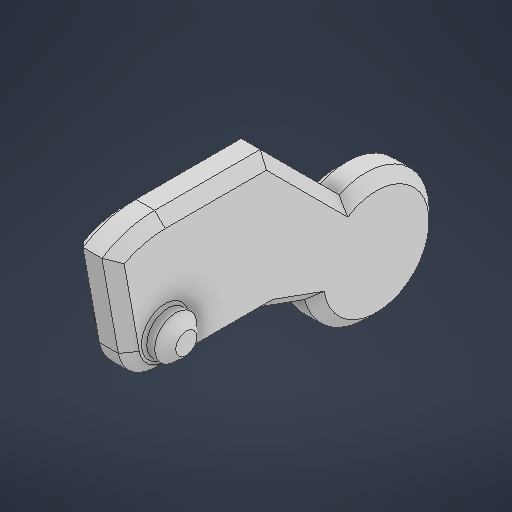
# Autodesk Inventor part: TrainPullert
Saved by Autodesk Inventor 2026.3 (Build 303398000, 398)
## iProperties
Created: 2026-05-02
Part Number: TrainPullert
Material: Generic
Document SubType Name: Modeling
Designer: frede
Density: 1 g/cm^3
Appearance: Default
Author: frede
Autodesk Inventor part; units mm, degrees
ref_plane "YZ Plane" through (0, 0, 0) normal (1, 0, 0) x (0, 1, 0)
ref_plane "XZ Plane" through (0, 0, 0) normal (0, 1, 0) x (-1, 0, 0)
ref_plane "XY Plane" through (0, 0, 0) normal (0, 0, 1) x (1, 0, 0)
sketch "Sketch1" plane through (0, 0, 0) normal (1, 0, 0) x (0, 1, 0)
  arc A0 (9.4, 0) -> (7.9599, 5) centre (0, 0) ccw
  circle A1 centre (0, 0) radius 3.5
  line L0 (-0.6243, 3.4439) -> (7.9599, 5)
  line L1 (-3.5, 0) -> (-3.5, -10)
  line L2 (9.4, 0) -> (9.4, -10)
  line L3 (-3.5, -10) -> (-5.0279, -14.1978)
  line L4 (-3.5, -10) -> (26.5, -10) construction
  line L5 (1.9372, -17.4628) -> (9.4, -10)
  arc A2 (-5.0279, -14.1978) -> (1.9372, -17.4628) centre (-3.5, -20) ccw
  dimension "d0" = 18.8
  dimension "d2" = 7
  dimension "d4" = 5
  dimension "d5" = 10
  dimension "d7" = 110
  dimension "d25" = 45
  dimension "d26" = 12
  constraints: 12 end point, 6 point on circle, 3 centre point, 3 tangent, 2 coincident, 2 vertical, 1 horizontal
  measures "d0" diameter of A0
  measures "d2" diameter of A1
  measures "d4" vertical distance of point (0, 0) L0.end
  measures "d5" distance of L2.start L2.end
  measures "d7" angle of L3 L4
  measures "d25" angle of L2 L5
  measures "d26" diameter of A2
extrude "Extrusion1" add sketch "Sketch1" along normal blind 3.8
sketch "Sketch2" plane through (3.8, 0, 0) normal (1, 0, 0) x (0, 0, -1)
  circle A0 centre (0, 0) radius 2
  dimension "d12" = 4
  constraints: 1 centre point, 1 coincident
  measures "d12" diameter of A0
extrude "Extrusion2" add sketch "Sketch2" along normal blind 2
sketch "Sketch3" plane through (0, 0, 0) normal (-1, 0, 0) x (0, 0, 1)
  circle A0 centre (0, 0) radius 2
  dimension "d15" = 4
  constraints: 1 centre point, 1 coincident
  measures "d15" diameter of A0
extrude "Extrusion3" add sketch "Sketch3" along normal blind 2
chamfer "Chamfer1" distance 1 angle 45 18 edges at (0, 9.4, -5) (0, 9.0328, 2.6016) (0, 3.6678, 4.2219) (0, -2.6865, 2.2433) (0, -3.5, -5) (0, -4.2639, -12.0989) (0, 5.6686, -13.7314) (3.8, 5.6686, -13.7314) (3.8, 9.4, -5) (3.8, 9.0328, 2.6016) (3.8, 3.6678, 4.2219) (3.8, -2.6865, 2.2433) (3.8, -3.5, -5) (3.8, -4.2639, -12.0989) (5.8, 0, 2) (-2, 0, -2) (3.8, -6.0467, -25.4327) (0, -6.0467, -25.4327)
fillet "Fillet1" radius 0.25 2 edges at (3.8, 0, 2) (0, 0, -2)
body "Solid1"
